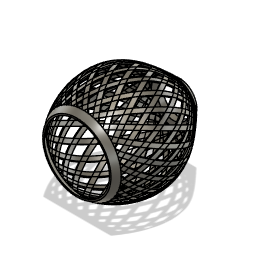
Lampshed v1 (Autodesk Fusion 360 design; units mm, degrees)
Autodesk Fusion 360 part; units mm, degrees
sketch "Sketch1" plane through (0, 0, 0) normal (0, 1, 0) x (1, 0, 0)
  line L0 (0, 0) -> (0, 135)
  line L1 (0, 135) -> (-23.4, 135)
  line L2 (0, 0) -> (-45, 0)
  spline S0 degree 5 poles (-45, 0) (-47.5993, 3.5621) (-52.3606, 10.5946) (-58.1904, 20.8687) (-63.4771, 33.9628) (-66.638, 49.0494) (-67.1343, 62.5896) (-65.6119, 74.4925) (-62.3934, 85.0212) (-57.278, 95.0464) (-49.7088, 105.7762) (-41.122, 115.9291) (-32.9661, 124.8874) (-26.723, 131.5192) (-23.4, 135) knots 0 0 0 0 0 0 0.1 0.2 0.3 0.4 0.5 0.6 0.7 0.8 0.9 1 1 1 1 1 1
  line L3 (-40.4345, 117.1564) -> (-6.3655, 152.8436)
  line L4 (-32.4292, -17.2267) -> (-57.5708, 17.2267)
  point P0 (-65, 75)
  dimension "d1" = 135
  dimension "d2" = 23.4
  dimension "d3" = 45
  constraint coincident L0.start L2.start
  constraint vertical L0
  constraint perpendicular L0 L1
  constraint perpendicular L0 L2
  constraint midpoint L1.end L3
  constraint midpoint L2.end L4
  measures "d1" distance of L0.start L0.end
  measures "d2" distance of L0.end L1.end
  measures "d3" distance of L0.start L2.end
revolve "Revolve1" add sketch "Sketch1" angle 360 about axis through (0, 0, 0) along (0, 0, -1) makes body 1
ref_plane "WorkPlane1" through (0, 0, -127) normal (0, 0, -1) x (-1, 0, 0)
split "Split1" by plane through (0, 0, -127) normal (0, 0, -1) bodies 1 makes body 2 at (-2.2493, -28.4375, -129.5826)
sketch "Sketch2" plane through (0, 0, -135) normal (0, 0, -1) x (-1, 0, 0)
  circle A0 centre (0, 0) radius 23.4
  circle A1 centre (0, 0) radius 21
  dimension "d6" = 42
  constraint concentric A0 A1
  measures "d6" diameter of A1
extrude "Extrude1" cut sketch "Sketch2" against normal up to surface (8 mm away) contours A1 bodies 2
shell "Shell1" thickness 1.6 removed faces 2 at (-8.8535, 9.5418, 0) at (-3.049, 8.8374, -127) on bodies 1
ref_plane "WorkPlane2" through (0, 0, -8) normal (0, 0, 1) x (1, 0, 0)
split "Split2" by plane through (0, 0, -8) normal (0, 0, 1) bodies 1 makes body 3 at (40.6354, -23.4553, -2.6878)
sketch "Sketch3" plane through (0, 0, 0) normal (0, 1, 0) x (1, 0, 0)
  line L0 (30.9347, 127) -> (-30.9347, 127)
  line L1 (-50.4566, 8) -> (50.4566, 8)
  spline S0 degree 3 poles (30.9347, 127) (39.8091, 117.433) (46.4735, 109.6906) (56.5156, 96.0464) (59.943, 90.0802) (64.7413, 77.5561) (66.1661, 70.9538) (66.9783, 55.8382) (66.3075, 47.3457) (61.4803, 28.822) (57.2731, 18.8257) (50.5951, 8.2189) (50.526, 8.1095) (50.4566, 8) knots -0.951849 -0.951849 -0.951849 -0.951849 -0.770569 -0.770569 -0.58929 -0.58929 -0.409899 -0.409899 -0.22862 -0.22862 -0.047341 -0.047341 -0.045452 -0.045452 -0.045452 -0.045452
  spline S1 degree 3 poles (-30.9347, 127) (-39.8091, 117.433) (-46.4735, 109.6906) (-56.5156, 96.0464) (-59.943, 90.0802) (-64.7413, 77.5561) (-66.1661, 70.9538) (-66.9783, 55.8382) (-66.3075, 47.3457) (-61.4803, 28.822) (-57.2731, 18.8257) (-50.5951, 8.2189) (-50.526, 8.1095) (-50.4566, 8) knots -0.951849 -0.951849 -0.951849 -0.951849 -0.770569 -0.770569 -0.58929 -0.58929 -0.409899 -0.409899 -0.22862 -0.22862 -0.047341 -0.047341 -0.045452 -0.045452 -0.045452 -0.045452
  line L2 (-27.548, 127) -> (26.3639, 8)
  line L3 (-21.548, 127) -> (32.3639, 8)
  dimension "d11" = 6
  constraint coincident L0 L2.start
  constraint coincident L1 L2.end
  constraint coincident L0 L3.start
  constraint coincident L1 L3.end
  constraint parallel L2 L3
  measures "d11" distance of L2.start L3.start
extrude "Extrude2" cut sketch "Sketch3" along normal mid plane 160 contours L0 L1 L2 L3 keep common part bodies 1 makes body 4 at (26.0137, -45.0372, -13.6697)
pattern_circular "C-Pattern1" count 22 over 360 about axis through (0, 0, 1.75) along (0, 0, 1) of bodies 1 makes body 5 at (12.2725, 50.5406, -13.6681) makes body 6 at (-2.471, 51.9559, -13.6773) makes body 7 at (-16.9955, 49.1511, -13.6631) makes body 8 at (-30.1053, 42.3711, -13.6123) makes body 9 at (-40.8703, 32.1601, -13.6628) makes body 10 at (-48.278, 19.3412, -13.6661) makes body 11 at (-51.7754, 4.9519, -13.6722) makes body 12 at (-51.0754, -9.84, -13.6773) makes body 13 at (-46.2285, -23.7955, -13.6402) makes body 14 at (-37.6518, -35.8572, -13.6417) makes body 15 at (-26.0137, -45.0372, -13.6697) makes body 16 at (-12.2725, -50.5406, -13.6681) makes body 17 at (2.471, -51.9559, -13.6773) makes body 18 at (16.9955, -49.1511, -13.6631) makes body 19 at (30.1053, -42.3711, -13.6123) makes body 20 at (40.8703, -32.1601, -13.6628) makes body 21 at (48.278, -19.3412, -13.6661) makes body 22 at (51.7754, -4.9519, -13.6722) makes body 23 at (51.0754, 9.84, -13.6773) makes body 24 at (46.2285, 23.7955, -13.6402) makes body 25 at (37.6518, 35.8572, -13.6417)
pattern_circular "C-Pattern2" count 22 over 360 about axis through (0, 0, 1.75) along (0, 0, 1) of bodies 4 makes body 26 at (37.6518, -35.8572, -13.6417) makes body 27 at (46.2285, -23.7955, -13.6402) makes body 28 at (51.0754, -9.84, -13.6773) makes body 29 at (51.7754, 4.9519, -13.6722) makes body 30 at (48.278, 19.3412, -13.6661) makes body 31 at (40.8703, 32.1601, -13.6628) makes body 32 at (30.1053, 42.3711, -13.6123) makes body 33 at (16.9955, 49.1511, -13.6631) makes body 34 at (2.471, 51.9559, -13.6773) makes body 35 at (-12.2725, 50.5406, -13.6681) makes body 36 at (-26.0137, 45.0372, -13.6697) makes body 37 at (-37.6518, 35.8572, -13.6417) makes body 38 at (-46.2285, 23.7955, -13.6402) makes body 39 at (-51.0754, 9.84, -13.6773) makes body 40 at (-51.7754, -4.9519, -13.6722) makes body 41 at (-48.278, -19.3412, -13.6661) makes body 42 at (-40.8703, -32.1601, -13.6628) makes body 43 at (-30.1053, -42.3711, -13.6123) makes body 44 at (-16.9955, -49.1511, -13.6631) makes body 45 at (-2.471, -51.9559, -13.6773) makes body 46 at (12.2725, -50.5406, -13.6681)
